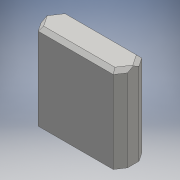
# Autodesk Inventor part: Frame2
Saved by Autodesk Inventor 2016 (Build 200138000, 138)
## iProperties
Created: 2017-07-01
Part Number: Frame2
Material: Generic
Document SubType Name: Modeling
Designer: ALIREZA
Density: 1 g/cm^3
Appearance: Default
Author: ALIREZA
Autodesk Inventor part; units mm, degrees
ref_plane "YZ Plane" through (0, 0, 0) normal (1, 0, 0) x (0, 1, 0)
ref_plane "XZ Plane" through (0, 0, 0) normal (0, 1, 0) x (-1, 0, 0)
ref_plane "XY Plane" through (0, 0, 0) normal (0, 0, 1) x (1, 0, 0)
sketch "Sketch1" plane through (0, 0, 0) normal (0, 0, 1) x (1, 0, 0)
  line L0 (-52.5, -20) -> (52.5, -20)
  line L1 (52.5, 20) -> (-52.5, 20)
  line L2 (-52.5, -20) -> (52.5, 20) construction
  line L3 (52.5, -20) -> (-52.5, 20) construction
  line L4 (-50, 17.5) -> (50, 17.5)
  line L5 (50, -17.5) -> (-50, -17.5)
  line L6 (-50, 17.5) -> (50, -17.5) construction
  line L7 (50, 17.5) -> (-50, -17.5) construction
  line L8 (60.5, 0) -> (60.5, 8)
  line L9 (60.5, 8) -> (52.5, 20)
  line L10 (60.5, 0) -> (60.5, -8)
  line L11 (60.5, -8) -> (52.5, -20)
  line L12 (50, -17.5) -> (56.5426, -7.6861)
  line L13 (56.5426, -7.6861) -> (56.5426, 7.6861)
  line L14 (56.5426, 7.6861) -> (50, 17.5)
  line L15 (0, 0) -> (0, 38.4543) construction
  line L16 (-60.5, 0) -> (-60.5, 8)
  line L17 (-60.5, 8) -> (-52.5, 20)
  line L18 (-60.5, 0) -> (-60.5, -8)
  line L19 (-60.5, -8) -> (-52.5, -20)
  line L20 (-50, -17.5) -> (-56.5426, -7.6861)
  line L21 (-56.5426, -7.6861) -> (-56.5426, 7.6861)
  line L22 (-56.5426, 7.6861) -> (-50, 17.5)
  dimension "d0" = 105
  dimension "d1" = 40
  dimension "d2" = 100
  dimension "d3" = 35
  dimension "d5" = 8
  dimension "d6" = 8
  constraints: 46 end point, 5 parallel, 5 symmetric about line, 4 midpoint, 2 horizontal, 2 point on line, 1 vertical
  measures "d0" distance of L1.end L1.start
  measures "d1" distance of L1.start L0.end
  measures "d2" distance of L5.start L5.end
  measures "d3" distance of L4.end L5.start
  measures "d5" distance of L8.start L8.end
  measures "d6" distance of L8.start L10.end
extrude "Extrusion1" add sketch "Sketch1" along normal blind 120
sketch "Sketch2" plane through (0, 0, 120) normal (0, 0, 1) x (1, 0, 0)
  line L0 (-56.5426, 7.6861) -> (-50, 17.5) projected
  line L1 (-50, 17.5) -> (50, 17.5) projected
  line L2 (50, 17.5) -> (56.5426, 7.6861) projected
  line L3 (56.5426, 7.6861) -> (56.5426, -7.6861) projected
  line L4 (56.5426, -7.6861) -> (50, -17.5) projected
  line L5 (50, -17.5) -> (-50, -17.5) projected
  line L6 (-50, -17.5) -> (-56.5426, -7.6861) projected
  line L7 (-56.5426, -7.6861) -> (-56.5426, 7.6861) projected
  point P0 (0, 0)
extrude "Extrusion2" add sketch "Sketch2" against normal blind 2.5
sketch "Sketch3" plane through (0, 0, 0) normal (0, 0, -1) x (-1, 0, 0)
  point P0 (0, 0)
fillet "Fillet1" radius 1 2 edges at (0, -17.5, 117.5) (0, 17.5, 117.5)
chamfer "Chamfer1" distance 5 angle 45 6 edges at (0, 20, 120) (-56.5, 14, 120) (-56.5, -14, 120) (0, -20, 120) (56.5, 14, 120) (56.5, -14, 120)
body "Solid1"
